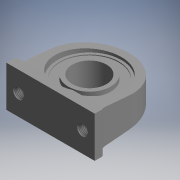
# Autodesk Inventor part: PDRUPN50_b
Saved by Autodesk Inventor 2017.3 (Build 213256000, 256)
## iProperties
Part Number: PDRUPN50_b
Material: Generic
Catalog Web Link: www.cadenas.de
Description: PDRUP,PDRUPN_body-Ball Bearing Units -Pillow Shaped Narrow Type-
Vendor: MISUMI
Document SubType Name: Modeling
Designer: partserver
Manufacturer: MISUMI
Mass: 404.952 g
Surface Area: 639.766 cm^2
Volume: 404.952 cm^3
Density: 1 g/cm^3
Appearance: PSOLRGB-175-175-175
Category: PARTsolutions
Company: MISUMI
Title: PDRUPN50
Author: Cadenas PARTsolutions
Comments: Ball Bearing Units -Pillow Shaped Narrow Type-
PSOL_IDENT_0: {$CADENAS_DATA\23d-libs\misumi\metric\12_bearing_holders\pdrup\pdrup_body.prj},172 {VTYP=3D},{NB=PDR
PSOL_IDENT_1: UPN50_b},{LINA=PDRUPN50},{NN=PDRUP,PDRUPN_body},{DATE=13.11.2019 02:15:11},{GEOMDATE=11.11.2019 09:0
PSOL_IDENT_2: 8:53},{VERSION=},{LINEID=100},{WBVAR=TS},{WBNUMERIC=}  {NB=PDRUPN50_b},{LINA=PDRUPN50},{KT=DUMMY},{P
PSOL_IDENT_3: N=PDRUPN50},{TYPE=PDRUPN},{MATH=Cast Iron Class No.30},{MATB=52100 Bearing Steel},{MATRS=Nitrile Rub
PSOL_IDENT_4: ber},{MATSS=4137 Alloy Steel},{PRECISION=JIS B 1558/JIS B 1514/JIS B 1559},{OT=-15 ~+100},{TS=2},{TS
PSOL_IDENT_5: ALG='1','Lubrication Type' , '2','Oil-Free Type'},{D=50},{JIS=UC210D1},{H=57.2},{L=130},{L1=94},{A=6
PSOL_IDENT_6: 0},{M=M16x2},{MD=16},{MPITCH=2.0},{TT=25},{T1=14},{H1=116},{B=51.6},{S=19.0},{CR=35.0},{COR=23.20},{
PSOL_IDENT_7: M1=M8x1},{M1D=8},{M1PITCH=1.00},{M1L=10},{MASS=2600},{RLD=58.8},{RLC=47.0},{LB1=86.48},{LB2=62.4},{L
PSOL_IDENT_8: D1=51},{LD2=33},{LD3=25},{LD4=27.5},{LD5=58.8},{NCL=1.5},{KCL=23.6},{R1=4},{R2=8.0}
NB: PDRUPN50_b
NN: PDRUP,PDRUPN_body
NT: Ball Bearing Units -Pillow Shaped Narrow Type-
NBSYN: $PN._b
LINA: PDRUPN50
CATALOG: Misumi
PN: PDRUPN50
TYPE: PDRUPN
MATH: Cast Iron Class No.30
MATB: 52100 Bearing Steel
MATRS: Nitrile Rubber
MATSS: 4137 Alloy Steel
PRECISION: JIS B 1558/JIS B 1514/JIS B 1559
OT: -15 ~+100
TS: Oil-Free Type
D: 50
JIS: UC210D1
H: 57.2
L: 130
L1: 94
A: 60
M: M16x2
TT: 25
H1: 116
B: 51.6
S: 19
CR: 35
COR: 23.2
M1: M8x1
MASS: 2600
SUPPLIER: MISUMI
ARTICLENO: PDRUPN50_b
BOMINFO: PDRUPN50
CREATOR: CADENAS GmbH
Autodesk Inventor part; units mm, degrees
sketch "_____3" plane through (0, 0, 0) normal (0, 0, 1) x (1, 0, 0)
  line L0 (-65, 10) -> (-65, 0)
  line L1 (-65, 0) -> (65, 0)
  line L2 (65, 0) -> (65, 10)
  arc A0 (65, 10) -> (62.9333, 13.5017) centre (61, 10) ccw
  arc A1 (58.8, 20.5052) -> (62.9333, 13.5017) centre (66.8, 20.5052) ccw
  line L3 (58.8, 20.5052) -> (58.8, 57.2)
  arc A2 (58.8, 57.2) -> (-58.8, 57.2) centre (0, 57.2) ccw
  line L4 (-58.8, 57.2) -> (-58.8, 20.5052)
  arc A3 (-62.9333, 13.5017) -> (-58.8, 20.5052) centre (-66.8, 20.5052) ccw
  arc A4 (-62.9333, 13.5017) -> (-65, 10) centre (-61, 10) ccw
  constraints: 10 end point, 10 point on circle, 5 centre point
extrude "Extrusion1" add sketch "_____3" along normal mid plane 60
sketch "_____4" plane through (0, 0, 0) normal (1, 0, 0) x (0, 0, -1)
  line L0 (16.5, 116) -> (25.5, 14)
  line L1 (25.5, 14) -> (30, 14)
  line L2 (30, 14) -> (30, 116)
  line L3 (30, 116) -> (16.5, 116)
  constraints: 8 end point
extrude "Extrusion2" cut sketch "_____4" along normal mid plane 140
sketch "_____5" plane through (0, 0, 0) normal (1, 0, 0) x (0, 0, -1)
  line L0 (-30, 14) -> (-25.5, 14)
  line L1 (-25.5, 14) -> (-16.5, 116)
  line L2 (-16.5, 116) -> (-30, 116)
  line L3 (-30, 116) -> (-30, 14)
  constraints: 8 end point
extrude "Extrusion3" cut sketch "_____5" along normal mid plane 140
sketch "_____7" plane through (0, 0, 0) normal (1, 0, 0) x (0, 0, -1)
  line L0 (30, 57.2) -> (12.5, 57.2)
  line L1 (12.5, 57.2) -> (12.5, 100.44)
  line L2 (12.5, 100.44) -> (13.75, 100.44)
  line L3 (13.75, 100.44) -> (13.75, 104.2)
  line L4 (13.75, 104.2) -> (30, 104.2)
  line L5 (30, 104.2) -> (30, 57.2)
  line L6 (30, 57.2) -> (12.5, 57.2)
  constraints: 14 end point
revolve "Revolution1" cut sketch "_____7" angle 360 about axis through (0, 57.2, -30) along (0, 0, -1)
sketch "_____8" plane through (0, 0, 0) normal (1, 0, 0) x (0, 0, -1)
  line L0 (-12.5, 57.2) -> (-30, 57.2)
  line L1 (-30, 57.2) -> (-30, 104.2)
  line L2 (-30, 104.2) -> (-13.75, 104.2)
  line L3 (-13.75, 104.2) -> (-13.75, 100.44)
  line L4 (-13.75, 100.44) -> (-12.5, 100.44)
  line L5 (-12.5, 100.44) -> (-12.5, 57.2)
  line L6 (-12.5, 57.2) -> (-30, 57.2)
  constraints: 14 end point
revolve "Revolution2" cut sketch "_____8" angle 360 about axis through (0, 57.2, 12.5) along (0, 0, -1)
sketch "_____9" plane through (0, 0, 0) normal (1, 0, 0) x (0, 0, -1)
  line L0 (19, 57.2) -> (-32.6, 57.2)
  line L1 (-32.6, 57.2) -> (-32.6, 88.4)
  line L2 (-32.6, 88.4) -> (19, 88.4)
  line L3 (19, 88.4) -> (19, 57.2)
  line L4 (19, 57.2) -> (-32.6, 57.2)
  constraints: 10 end point
revolve "Revolution3" add sketch "_____9" angle 360 about axis through (0, 57.2, -19) along (0, 0, -1)
sketch "Sketch7" plane through (0, 57.2, 32.6) normal (0, 0, 1) x (1, 0, 0)
  point P0 (0, 0)
hole "Hole1" at (0, 57.2, 32.6) direction (0, 0, -1) diameter 50 depth 61.6
sketch "Sketch8" plane through (-65, 0, 30) normal (0, -1, 0) x (1, 0, 0)
  point P0 (112, -30)
hole "Hole2" at (47, 0, 0) direction (0, 1, 0) diameter 13.835 depth 31 tip angle 120 countersink diameter 16 countersink angle 90 thread size "M16x2" class "6H" standard "ISO Metric profile"
sketch "Sketch9" plane through (-65, 0, 30) normal (0, -1, 0) x (1, 0, 0)
  point P0 (18, -30)
hole "Hole3" at (-47, 0, 0) direction (0, 1, 0) diameter 13.835 depth 31 tip angle 120 countersink diameter 16 countersink angle 90 thread size "M16x2" class "6H" standard "ISO Metric profile"
sketch "_____13" plane through (0, 0, 0) normal (1, 0, 0) x (0, 0, -1)
  line L0 (-23.6, 57.2) -> (-23.6, 88.4)
  line L1 (-23.6, 88.4) -> (-19.6, 88.4)
  line L2 (-19.6, 88.4) -> (-20.1415, 87.8585)
  line L3 (-20.1415, 87.8585) -> (-20.1415, 57.2)
  line L4 (-20.1415, 57.2) -> (-23.6, 57.2)
  line L5 (-23.6, 57.2) -> (-23.6, 88.4)
  constraints: 12 end point
revolve "Revolution4" cut sketch "_____13" angle 360 about axis through (0, 57.2, 23.6) along (0, -1, 0)
thread "Thread1" size "M8x1" class "6H" standard "ISO Metric profile" length 5.6585
sketch "_____14" plane through (0, 0, 23.6) normal (0, 0, 1) x (1, 0, 0)
  line L0 (0, 57.2) -> (-27.02, 41.6)
  line L1 (-27.02, 41.6) -> (-29.02, 45.0641)
  line L2 (-29.02, 45.0641) -> (-28.2803, 44.8659)
  line L3 (-28.2803, 44.8659) -> (-1.7292, 60.1951)
  line L4 (-1.7292, 60.1951) -> (0, 57.2)
  line L5 (0, 57.2) -> (-27.02, 41.6)
  constraints: 12 end point
revolve "Revolution5" cut sketch "_____14" angle 360 about axis through (0, 57.2, 23.6) along (0.8660254, 0.5, 0)
thread "Thread2" size "M8x1" class "6H" standard "ISO Metric profile" length 5.6585
ref_plane "cp1_XY" through (0, 82.2, 23.6) normal (0, 1, 0) x (1, 0, 0)
ref_plane "cp1_YZ" through (0, 82.2, 23.6) normal (1, 0, 0) x (0, 0, -1)
ref_plane "cp1_ZX" through (0, 82.2, 23.6) normal (0, 0, -1) x (0, 1, 0)
ref_plane "cp2_XY" through (-21.6506, 44.7, 23.6) normal (-0.8660254, -0.5, 0) x (-0.5, 0.8660254, 0)
ref_plane "cp2_YZ" through (-21.6506, 44.7, 23.6) normal (-0.5, 0.8660254, 0) x (0, 0, -1)
ref_plane "cp2_ZX" through (-21.6506, 44.7, 23.6) normal (0, 0, -1) x (-0.8660254, -0.5, 0)
body "Solid1"
